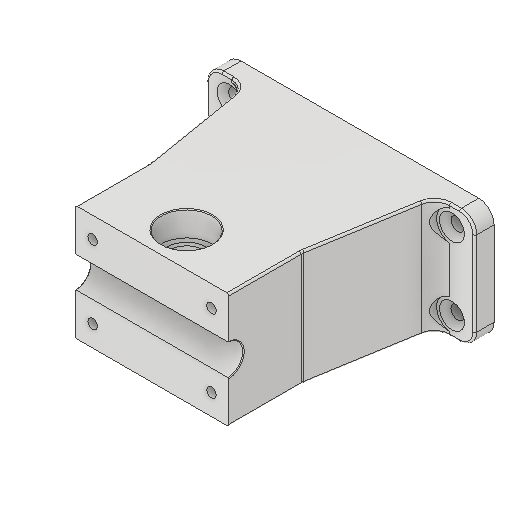
# Autodesk Inventor part: 3DP_PLA_Y_axis_linear_shaft_mount_front
Saved by Autodesk Inventor 2026.1 (Build 301233000, 233)
## iProperties
Created: 2018-06-17
Part Number: 3DP_PLA_Y_axis_linear_shaft_mount_front
Material: ABS Plastic
Document SubType Name: Modeling
Designer: Andrzej
Density: 1.06 g/cm^3
Appearance: Smooth - White
Author: Andrzej
Autodesk Inventor part; units mm, degrees
ref_plane "YZ Plane" through (0, 0, 0) normal (1, 0, 0) x (0, 1, 0)
ref_plane "XZ Plane" through (0, 0, 0) normal (0, 1, 0) x (-1, 0, 0)
ref_plane "XY Plane" through (0, 0, 0) normal (0, 0, 1) x (1, 0, 0)
sketch "Sketch1" plane through (0, 0, 0) normal (0, 0, 1) x (1, 0, 0)
  line L0 (-12.9235, 18.928) -> (27.0765, 18.928)
  line L1 (27.0765, 18.928) -> (27.0765, -11.072)
  line L2 (27.0765, -11.072) -> (-12.9235, -11.072)
  line L3 (-12.9235, -11.072) -> (-12.9235, 18.928)
  line L4 (27.0765, -11.072) -> (42.0765, -11.072)
  line L5 (42.0765, -11.072) -> (42.0765, 18.928)
  line L6 (42.0765, 18.928) -> (27.0765, 18.928)
  line L7 (-12.9235, 18.928) -> (-27.9235, 18.928)
  line L8 (-12.9235, -11.072) -> (-27.9235, -11.072)
  line L9 (-27.9235, -11.072) -> (-27.9235, 18.928)
  point P0 (0, 0)
  point P1 (36.0765, -6.072)
  point P2 (36.0765, 13.928)
  point P3 (-21.9235, -6.072)
  point P4 (-21.9235, 13.928)
  dimension "d1" = 30
  dimension "d48" = 15
  dimension "d49" = 15
  dimension "d50" = 6
  dimension "d51" = 6
  dimension "d52" = 40
  dimension "d53" = 5
  dimension "d54" = 5
  constraints: 20 end point, 4 perpendicular, 3 horizontal, 2 horizontal alignment, 2 parallel, 2 vertical alignment, 1 point on line
  measures "d1" distance of L0.end L1.end
  measures "d48" distance of L1.end L4.end
  measures "d49" distance of L2.end L8.end
  measures "d50" distance from line of L5 point (36.076, -6.072)
  measures "d51" distance from line of L9 point (-21.924, -6.072)
  measures "d52" distance between parallel lines of L3 L1
  measures "d53" distance from line of L4 point (36.076, -6.072)
  measures "d54" distance from line of L6 point (36.076, 13.928)
extrude "Extrusion1" add sketch "Sketch1" along normal blind 49.2 contours L0 L1 L2 L3
extrude "Extrusion2" add sketch "Sketch1" against normal blind 5
hole "Hole1" at (36.0765, -6.072, 0) at (36.0765, 13.928, 0) at (-21.9235, 13.928, 0) at (-21.9235, -6.072, 0) direction (0, 0, -1) diameter 3.5 end through all
sketch "Sketch2" plane through (27.0765, -11.072, 49.2) normal (1, 0, 0) x (0, 0, -1)
  line L0 (49.2, 30) -> (0, 30) projected
  line L1 (0, 0) -> (0, 30) projected
  line L2 (49.2, 0) -> (0, 0) projected
  circle A0 centre (-0.2, 15) radius 4.025
  line L3 (49.2, 30) -> (49.2, 0) projected
  dimension "d20" = 30
  dimension "d21" = 15
  dimension "d22" = 0.2
  dimension "d23" = 8.05
  constraints: 1 centre point, 1 coincident
  measures "d20" distance between parallel lines of L0 L2
  measures "d21" distance from line of L2 point (-0.2, 15)
  measures "d22" distance from line of L1 point (-0.2, 15)
  measures "d23" diameter of A0
extrude "Extrusion3" cut sketch "Sketch2" against normal through all contours A0 L1 | L1 A0
sketch "Sketch3" plane through (0, 0, 49.2) normal (0, 0, 1) x (1, 0, 0)
  line L0 (27.0765, -0.092) -> (-12.9235, -0.092) projected
  line L1 (-12.9235, -0.092) -> (-12.9235, -11.072) projected
  line L2 (-12.9235, -11.072) -> (27.0765, -11.072) projected
  line L3 (27.0765, -11.072) -> (27.0765, -0.092) projected
  line L4 (-12.9235, 7.948) -> (27.0765, 7.948) projected
  line L5 (27.0765, 7.948) -> (27.0765, 18.928) projected
  line L6 (27.0765, 18.928) -> (-12.9235, 18.928) projected
  line L7 (-12.9235, 18.928) -> (-12.9235, 7.948) projected
  point P0 (0, 0)
  point P1 (22.5765, -5.582)
  point P2 (-8.4235, -5.582)
  point P3 (22.5765, 13.438)
  point P4 (-8.4235, 13.438)
  dimension "d26" = 4.5
  dimension "d27" = 10.98
  dimension "d28" = 5.49
  dimension "d29" = 5.49
  dimension "d30" = 4.5
  constraints: 2 horizontal alignment, 2 vertical alignment
  measures "d26" distance from line of L3 point (22.576, -5.582)
  measures "d27" distance between parallel lines of L0 L2
  measures "d28" distance from line of L2 point (22.576, -5.582)
  measures "d29" distance from line of L6 point (22.576, 13.438)
  measures "d30" distance from line of L1 point (-8.424, -5.582)
hole "Hole2" at (22.5765, -5.582, 49.2) at (-8.4235, -5.582, 49.2) at (22.5765, 13.438, 49.2) at (-8.4235, 13.438, 49.2) direction (0, 0, -1) diameter 2.5 depth 20 tip angle 118
sketch "Sketch6" plane through (-12.9235, 18.928, 49.2) normal (0, 1, 0) x (1, 0, 0)
  line L0 (0, 49.2) -> (0, 0) projected
  line L1 (40, 0) -> (0, 0) projected
  line L2 (40, 49.2) -> (40, 0) projected
  line L3 (55, 49.2) -> (40, 49.2) projected
  line L4 (55, 49.2) -> (55, 54.2) projected
  line L5 (-15, 54.2) -> (55, 54.2) projected
  line L6 (-15, 49.2) -> (-15, 54.2) projected
  line L7 (0, 49.2) -> (-15, 49.2) projected
  circle A0 centre (20, 9) radius 6.575
  dimension "d55" = 13.15
  dimension "d56" = 40
  dimension "d57" = 20
  dimension "d58" = 9
  constraints: 1 centre point
  measures "d55" diameter of A0
  measures "d56" distance of L1.start L0.end
  measures "d57" distance from line of L2 A0.centre
  measures "d58" distance from line of L1 A0.centre
extrude "Extrusion4" cut sketch "Sketch6" against normal blind 6.5 contours A0
hole "Hole4" at (7.0765, 18.928, 40.2) direction (0, -1, 0) diameter 6.5 end through all
sketch "Sketch7" plane through (-12.9235, -11.072, 49.2) normal (0, -1, 0) x (1, 0, 0)
  circle A0 centre (20, -9) radius 6.575 projected
  point P0 (12.9235, -49.2)
extrude "Extrusion5" cut sketch "Sketch7" against normal blind 4
chamfer "Chamfer1" distance 1.5 angle 45 2 edges at (7.0765, 12.428, 36.95) (7.0765, -7.072, 36.95)
chamfer "Chamfer2" distance 0.2 angle 45 4 edges at (0.5015, 18.928, 40.2) (0.5015, -11.072, 40.2) (-12.9235, 3.928, 45.375) (27.0765, 3.928, 45.375)
fillet "Fillet3" radius 4 4 edges at (-27.9235, 18.928, -2.5) (-27.9235, -11.072, -2.5) (42.0765, 18.928, -2.5) (42.0765, -11.072, -2.5)
chamfer "Chamfer3" distance 5 distance2 30 1 edges at (27.0765, 3.928, 0) measured on face at (29.5964, 0.9261, 0)
chamfer "Chamfer4" distance 5 distance2 30 1 edges at (-12.9235, 3.928, 0) measured on face at (-15.4434, 0.9261, 0)
fillet "Fillet5" radius 4 4 edges at (32.0765, 3.928, 0) (-17.9235, 3.928, 0) (27.0765, 3.928, 30) (-12.9235, 3.928, 30)
sketch "Sketch10" plane through (0, 0, 0) normal (0, 0, 1) x (1, 0, 0)
  line L0 (-21.312, 12.2883) -> (-21.312, -4.4323) projected
  arc A0 (-21.312, 15.5677) -> (-21.312, 12.2883) centre (-21.9235, 13.928) ccw projected
  line L1 (-21.312, 18.928) -> (-21.312, 15.5677) projected
  line L2 (-21.312, 18.928) -> (-23.9235, 18.928) projected
  arc A1 (-23.9235, 18.928) -> (-27.9235, 14.928) centre (-23.9235, 14.928) ccw projected
  line L3 (-27.9235, 14.928) -> (-27.9235, -7.072) projected
  arc A2 (-27.9235, -7.072) -> (-23.9235, -11.072) centre (-23.9235, -7.072) ccw projected
  line L4 (-23.9235, -11.072) -> (-21.312, -11.072) projected
  line L5 (-21.312, -7.7117) -> (-21.312, -11.072) projected
  arc A3 (-21.312, -4.4323) -> (-21.312, -7.7117) centre (-21.9235, -6.072) ccw projected
  line L6 (35.465, -4.4323) -> (35.465, 12.2883) projected
  arc A4 (35.465, -7.7117) -> (35.465, -4.4323) centre (36.0765, -6.072) ccw projected
  line L7 (35.465, -11.072) -> (35.465, -7.7117) projected
  line L8 (35.465, -11.072) -> (38.0765, -11.072) projected
  arc A5 (38.0765, -11.072) -> (42.0765, -7.072) centre (38.0765, -7.072) ccw projected
  line L9 (42.0765, -7.072) -> (42.0765, 14.928) projected
  arc A6 (42.0765, 14.928) -> (38.0765, 18.928) centre (38.0765, 14.928) ccw projected
  line L10 (38.0765, 18.928) -> (35.465, 18.928) projected
  line L11 (35.465, 15.5677) -> (35.465, 18.928) projected
  arc A7 (35.465, 12.2883) -> (35.465, 15.5677) centre (36.0765, 13.928) ccw projected
  point P0 (0, 0)
hole "Hole6" at (36.0765, -6.072, 0) at (36.0765, 13.928, 0) at (-21.9235, -6.072, 0) at (-21.9235, 13.928, 0) direction (0, 0, 1) diameter 8 end through all
fillet "Fillet6" radius 0.5 22 edges at (32.8795, 18.928, 0.9479) (27.0765, 18.928, 39.7655) (36.7707, 18.928, 0) (40.9049, 17.7564, 0) (42.0765, 3.928, 0) (40.9049, -9.9004, 0) (36.7707, -11.072, 0) (32.8795, -11.072, 0.9479) (29.3252, -11.072, 16.5079) (27.0765, -11.072, 39.7655) (29.3252, 18.928, 16.5079) (-18.7265, 18.928, 0.9479) (-22.6178, 18.928, 0) (-26.7519, 17.7564, 0) (-27.9235, 3.928, 0) (-26.7519, -9.9004, 0) (-22.6178, -11.072, 0) (-18.7265, -11.072, 0.9479) (-15.1722, -11.072, 16.5079) (-12.9235, -11.072, 39.7655) (-12.9235, 18.928, 39.7655) (-15.1722, 18.928, 16.5079)
chamfer "Chamfer5" distance 1.5 angle 45 4 edges at (36.0765, -4.322, 0) (36.0765, 15.678, 0) (-21.9235, -4.322, 0) (-21.9235, 15.678, 0)
fillet "Fillet7" radius 1 2 edges at (7.0765, -7.072, 35.45) (7.0765, 12.428, 35.45)
equation "\"d49\" = d48"
equation "\"d51\" = d50"
equation "\"d54\" = d53"
equation "\"d21\" = 0.5 * d20"
equation "\"d28\" = 0.5 * d27"
equation "\"d29\" = d28"
equation "\"d30\" = d26"
equation "\"d57\" = 0.5 * d56"
body "Solid1"
